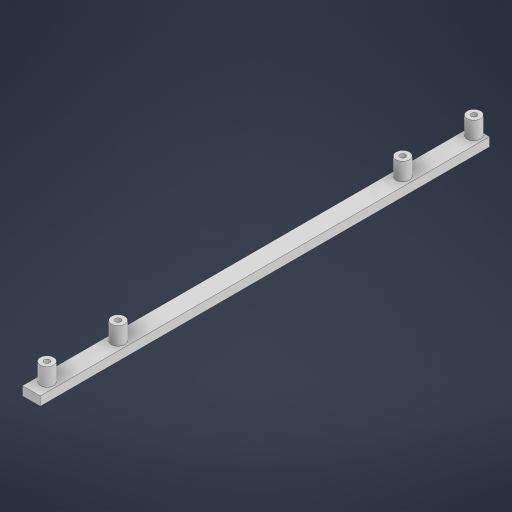
# Autodesk Inventor part: crossbrace_jig
Saved by Autodesk Inventor 2024 (Build 280153000, 153)
## iProperties
Created: 2023-11-10
Part Number: crossbrace_jig
Material: Generic
Document SubType Name: Modeling
Designer: avere
Density: 1 g/cm^3
Appearance: Default
Author: avere
Autodesk Inventor part; units mm, degrees
ref_plane "YZ Plane" through (0, 0, 0) normal (1, 0, 0) x (0, 1, 0)
ref_plane "XZ Plane" through (0, 0, 0) normal (0, 1, 0) x (-1, 0, 0)
ref_plane "XY Plane" through (0, 0, 0) normal (0, 0, 1) x (1, 0, 0)
sketch "Sketch1" plane through (0, 0, 0) normal (0, 0, 1) x (1, 0, 0)
  line L0 (3.175, 0) -> (3.175, 3.175)
  line L1 (3.175, 3.175) -> (-3.175, 3.175)
  line L2 (-3.175, 3.175) -> (-3.175, 0)
  line L3 (6.35, 0) -> (6.35, 6.35)
  line L4 (6.35, 6.35) -> (-6.35, 6.35)
  line L5 (-6.35, 6.35) -> (-6.35, 0)
  line L6 (-6.35, 0) -> (-3.175, 0)
  line L7 (3.175, 0) -> (6.35, 0)
  point P0 (0, 0)
  constraints: 16 end point, 4 parallel, 2 horizontal, 2 perpendicular
extrude "Extrusion1" add sketch "Sketch1" along normal blind 314.325
sketch "Sketch2" plane through (-6.35, 6.35, 0) normal (0, 1, 0) x (1, 0, 0)
  circle A0 centre (6.35, -4.7625) radius 1.985
  circle A1 centre (6.35, -55.5625) radius 1.985
  circle A2 centre (6.35, -309.5625) radius 1.985
  circle A3 centre (6.35, -258.7625) radius 1.985
  point P0 (6.35, 0)
  dimension "d2" = 3.97
  dimension "d3" = 3.97
  dimension "d4" = 3.97
  dimension "d5" = 3.97
  constraints: 4 centre point
  measures "d2" diameter of A0
  measures "d3" diameter of A1
  measures "d4" diameter of A2
  measures "d5" diameter of A3
extrude "Extrusion2" cut sketch "Sketch2" against normal blind 314.325
sketch "Sketch3" plane through (-6.35, 6.35, 0) normal (0, 1, 0) x (1, 0, 0)
  circle A0 centre (6.35, -4.7625) radius 1.985 projected
  circle A1 centre (6.35, -55.5625) radius 1.985 projected
  circle A2 centre (6.35, -258.7625) radius 1.985 projected
  circle A3 centre (6.35, -309.5625) radius 1.985 projected
  circle A4 centre (6.35, -4.7625) radius 4.7625
  circle A5 centre (6.35, -55.5625) radius 4.7625
  circle A6 centre (6.35, -258.7625) radius 4.7625
  circle A7 centre (6.35, -309.5625) radius 4.7625
  point P0 (6.35, 0)
  constraints: 4 coincident, 3 centre point, 1 vertical alignment, 2 other
extrude "Extrusion3" add sketch "Sketch3" along normal blind 12.7
sketch "Sketch4" plane through (0, 0, 314.325) normal (0, 0, 1) x (1, 0, 0)
  line L0 (-6.35, 0) -> (-3.175, 0) projected
  line L1 (-6.35, 0) -> (6.35, 0)
  line L2 (6.35, 0) -> (6.35, 6.35)
  line L3 (6.35, 6.35) -> (-6.35, 6.35)
  line L4 (-6.35, 6.35) -> (-6.35, 0)
  point P0 (0, 0)
  constraints: 8 end point, 2 parallel, 1 horizontal, 1 perpendicular
extrude "Extrusion4" add sketch "Sketch4" along normal blind 6.35
body "Solid1"
